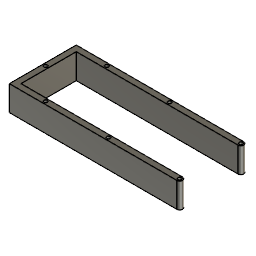
Belt Drive Arm (Autodesk Fusion 360 archive; units mm, degrees)
design "Wall"
Autodesk Fusion 360 part; units mm, degrees
sketch "Sketch1" plane through (0, 0, 0) normal (0, 0, 1) x (1, 0, 0)
  line L0 (0, 0) -> (160, 0)
  line L1 (0, 80) -> (160, 80)
  line L2 (0, 7) -> (160, 7)
  line L3 (160, 73) -> (0, 73)
  line L4 (0, 80) -> (-40, 80)
  line L5 (-40, 80) -> (-40, 0)
  line L6 (-40, 0) -> (0, 0)
  line L7 (0, 73) -> (-33, 73)
  line L8 (-33, 73) -> (-33, 7)
  line L9 (-33, 7) -> (0, 7)
  arc A0 (160, 73) -> (160, 80) centre (160, 76.5) ccw
  arc A1 (160, 0) -> (160, 7) centre (160, 3.5) ccw
  point P0 (0, 7)
  point P1 (0, 73)
  point P2 (160, 73)
  point P3 (160, 7)
  dimension "d1" = 160
  dimension "d2" = 80
  dimension "d3" = 7
  dimension "d4" = 7
  dimension "d5" = 7
  dimension "d6" = 7
  constraint coincident L0.start L6.end
  constraint horizontal L0
  constraint parallel L0 L1
  constraint coincident P0 L2.start
  constraint coincident P3 L2.end
  constraint parallel L0 L2
  constraint coincident P2 L3.start
  constraint coincident P1 L3.end
  constraint parallel L1 L4
  constraint perpendicular L1 L5
  constraint parallel L3 L7
  constraint perpendicular L2 L8
  constraint tangent L1 A0
  constraint tangent L0 A1
  measures "d1" distance of L0.start L0.end
  measures "d2" distance of L0 L1
  measures "d3" distance of L1.start P1
  measures "d4" distance of L0.start L2.start
  measures "d5" distance of L0.end P3
  measures "d6" distance of L1.end P2
extrude "Extrude1" add sketch "Sketch1" along normal blind 30
sketch "Sketch2" plane through (0, 0, 30) normal (0, 0, 1) x (-1, 0, 0)
  line L0 (40, 0) -> (-160, 0)
  line L1 (-160, -80) -> (40, -80)
  circle A0 centre (0, -3.5) radius 2.1
  circle A1 centre (0, -76.5) radius 2.1
  circle A2 centre (-160, -3.5) radius 2.1
  circle A3 centre (-160, -76.5) radius 2.1
  circle A4 centre (-75, -3.5) radius 2.1
  circle A5 centre (-75, -76.5) radius 2.1
  circle A6 centre (36.5, -40) radius 2.1
  line L2 (40, -80) -> (40, 0)
  line L3 (-160, -7) -> (33, -7)
  line L4 (33, -7) -> (33, -73)
  line L5 (33, -73) -> (-160, -73)
  arc A7 (-160, 0) -> (-160, -7) centre (-160, -3.5) ccw
  arc A8 (-160, -73) -> (-160, -80) centre (-160, -76.5) ccw
  point P0 (40, -40)
  point P1 (-75, -80)
  dimension "d9" = 4.2
  dimension "d10" = 4.2
  dimension "d11" = 4.2
  dimension "d12" = 4.2
  dimension "d13" = 4.2
  dimension "d14" = 4.2
  dimension "d15" = 4.2
  dimension "d21" = 3.5
  dimension "d22" = 3.5
  dimension "d23" = 3.5
  dimension "d24" = 3.5
  dimension "d28" = 85
  dimension "d29" = 85
  constraint coincident L1 P1
  measures "d9" diameter of A0
  measures "d10" diameter of A1
  measures "d11" diameter of A2
  measures "d12" diameter of A3
  measures "d13" diameter of A4
  measures "d14" diameter of A5
  measures "d15" diameter of A6
  measures "d21" distance of P0 A6.centre
  measures "d22" distance of L0 A0.centre
  measures "d23" distance of L0 A4.centre
  measures "d24" distance of L0 A2.centre
  measures "d28" horizontal distance of A3.centre P1
  measures "d29" horizontal distance of A2.centre P1
extrude "Extrude2" cut sketch "Sketch2" against normal blind 30 contours A0 | A1 | A2 | A3 | A4 | A5 | A6

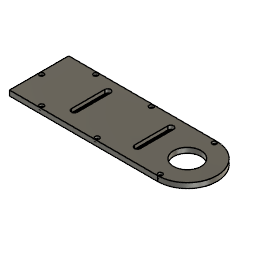
design "Top"
Autodesk Fusion 360 part; units mm, degrees
sketch "Sketch1" plane through (0, 0, 0) normal (0, 0, 1) x (1, 0, 0)
  line L0 (160, 80) -> (0, 80)
  line L1 (0, 0) -> (160, 0)
  arc A0 (160, 0) -> (160, 80) centre (160, 40) ccw
  line L2 (0, 80) -> (-40, 80)
  line L3 (-40, 80) -> (-40, 0)
  line L4 (-40, 0) -> (0, 0)
  dimension "d24" = 160
  dimension "d53" = 80
  constraint horizontal L0
  constraint coincident L1.start L4.end
  constraint tangent L1 A0
  constraint vertical L1.end L0.start
  constraint parallel L0 L2
  constraint perpendicular L2 L3
  measures "d24" distance of L1.start L1.end
  measures "d53" distance of L0 L1
extrude "Extrude1" add sketch "Sketch1" along normal blind 7
sketch "Sketch3" plane through (0, 0, 7) normal (0, 0, 1) x (-1, 0, 0)
  line L0 (40, 0) -> (-160, 0)
  line L1 (-160, -80) -> (40, -80)
  circle A0 centre (-75, -40) radius 3.05
  circle A1 centre (-75, -40) radius 5
  arc A2 (-160, 0) -> (-160, -80) centre (-160, -40) ccw
  line L2 (40, -80) -> (40, 0)
  point P0 (40, -40)
  dimension "d17" = 6.1
  dimension "d54" = 40
  dimension "d55" = 115
  constraint concentric A0 A1
  measures "d17" diameter of A0
  measures "d54" distance of L0 A0.centre
  measures "d55" distance of A0.centre P0
extrude "Extrude3" add sketch "Sketch3" against normal blind 8.7 contours A1
sketch "Sketch4" plane through (0, 0, 7) normal (0, 0, 1) x (-1, 0, 0)
  line L0 (40, 0) -> (-160, 0)
  line L1 (-160, -80) -> (40, -80)
  circle A0 centre (-160, -40) radius 18.5
  arc A1 (-160, 0) -> (-160, -80) centre (-160, -40) ccw
  line L2 (40, -80) -> (40, 0)
  point P0 (-200, -40)
  dimension "d25" = 37
  dimension "d56" = 40
  dimension "d57" = 40
  constraint midpoint A1 P0
  measures "d25" diameter of A0
  measures "d56" distance of L0 A0.centre
  measures "d57" distance of A0.centre P0
extrude "Extrude4" cut sketch "Sketch4" against normal blind 7 contours A0
sketch "Sketch7" plane through (0, 0, 7) normal (0, 0, 1) x (-1, 0, 0)
  circle A0 centre (-160, -40) radius 18.5
  arc A1 (-160, 0) -> (-160, -80) centre (-160, -40) ccw
  line L0 (-160, -80) -> (40, -80)
  line L1 (40, 0) -> (-160, 0)
  circle A2 centre (0, -76.5) radius 1.65
  circle A3 centre (0, -3.5) radius 1.65
  circle A4 centre (36.5, -40) radius 1.65
  circle A5 centre (-160, -76.5) radius 1.65
  circle A6 centre (-160, -3.5) radius 1.65
  circle A7 centre (-75, -3.5) radius 1.65
  circle A8 centre (-75, -76.5) radius 1.65
  line L2 (40, -80) -> (40, 0)
  point P0 (40, -40)
  point P1 (-75, -80)
  dimension "d58" = 3.3
  dimension "d59" = 3.3
  dimension "d60" = 3.3
  dimension "d62" = 3.3
  dimension "d63" = 3.3
  dimension "d64" = 3.3
  dimension "d65" = 3.3
  dimension "d66" = 3.5
  dimension "d68" = 3.5
  dimension "d69" = 3.5
  dimension "d70" = 3.5
  dimension "d73" = 3.5
  dimension "d86" = 3.5
  dimension "d87" = 85
  dimension "d88" = 85
  dimension "d106" = 40
  dimension "d107" = 3.5
  constraint coincident L0 P1
  measures "d58" diameter of A2
  measures "d59" diameter of A3
  measures "d60" diameter of A4
  measures "d62" diameter of A5
  measures "d63" diameter of A6
  measures "d64" diameter of A7
  measures "d65" diameter of A8
  measures "d66" distance of L0 A8.centre
  measures "d68" distance of L0 A5.centre
  measures "d69" distance of origin A3.centre
  measures "d70" distance of L1 A7.centre
  measures "d73" distance of P0 A4.centre
  measures "d86" distance of L1 A6.centre
  measures "d87" horizontal distance of A5.centre P1
  measures "d88" horizontal distance of A6.centre P1
  measures "d106" distance of A2.centre L2
  measures "d107" distance of L0 A2.centre
extrude "Extrude7" cut sketch "Sketch7" against normal blind 7 contours A2 | A3 | A4 | A5 | A6 | A7 | A8
sketch "Sketch8" plane through (0, 0, 7) normal (0, 0, 1) x (-1, 0, 0)
  circle A0 centre (-75, -76.5) radius 1.65
  circle A1 centre (-75, -3.5) radius 1.65
  circle A2 centre (36.5, -40) radius 1.65
  circle A3 centre (-160, -76.5) radius 1.65
  circle A4 centre (0, -3.5) radius 1.65
  circle A5 centre (-160, -40) radius 18.5
  arc A6 (-160, 0) -> (-160, -80) centre (-160, -40) ccw
  line L0 (-160, -80) -> (40, -80)
  line L1 (40, 0) -> (-160, 0)
  circle A7 centre (0, -76.5) radius 3
  circle A8 centre (36.5, -40) radius 3
  circle A9 centre (0, -3.5) radius 3
  circle A10 centre (-75, -76.5) radius 3
  circle A11 centre (-75, -3.5) radius 3
  circle A12 centre (-160, -76.5) radius 3
  circle A13 centre (-160, -3.5) radius 3
  circle A14 centre (-160, -3.5) radius 1.65
  line L2 (40, -80) -> (40, 0)
  circle A15 centre (0, -76.5) radius 1.65
  dimension "d76" = 6
  dimension "d77" = 6
  dimension "d78" = 6
  dimension "d79" = 6
  dimension "d80" = 6
  dimension "d81" = 6
  dimension "d82" = 6
  constraint concentric A7 A15
  constraint concentric A2 A8
  constraint concentric A4 A9
  constraint concentric A0 A10
  constraint concentric A1 A11
  constraint concentric A3 A12
  constraint concentric A13 A14
  measures "d76" diameter of A7
  measures "d77" diameter of A8
  measures "d78" diameter of A9
  measures "d79" diameter of A10
  measures "d80" diameter of A11
  measures "d81" diameter of A12
  measures "d82" diameter of A13
extrude "Extrude8" cut sketch "Sketch8" against normal blind 3 contours A7 | A8 | A9 | A10 | A11 | A12 | A13
sketch "Sketch9" plane through (0, 0, 7) normal (0, 0, 1) x (-1, 0, 0)
  circle A0 centre (-160, -76.5) radius 3
  circle A1 centre (36.5, -40) radius 3
  circle A2 centre (0, -3.5) radius 3
  circle A3 centre (-75, -76.5) radius 3
  circle A4 centre (-75, -3.5) radius 3
  circle A5 centre (-160, -3.5) radius 3
  circle A6 centre (-160, -40) radius 18.5
  arc A7 (-160, 0) -> (-160, -80) centre (-160, -40) ccw
  line L0 (-160, -80) -> (40, -80)
  line L1 (40, 0) -> (-160, 0)
  line L2 (-25, -20) -> (-25, -65)
  line L3 (-30.3, -20) -> (-30.3, -65)
  arc A8 (-30.3, -65) -> (-25, -65) centre (-27.65, -65) ccw
  arc A9 (-25, -20) -> (-30.3, -20) centre (-27.65, -20) ccw
  line L4 (-110, -20) -> (-110, -65)
  line L5 (-115.3, -20) -> (-115.3, -65)
  arc A10 (-110, -20) -> (-115.3, -20) centre (-112.65, -20) ccw
  arc A11 (-115.3, -65) -> (-110, -65) centre (-112.65, -65) ccw
  line L6 (40, -80) -> (40, 0)
  circle A12 centre (0, -76.5) radius 3
  point P0 (40, -40)
  point P1 (-160, -40)
  point P2 (-75, -40)
  dimension "d89" = 45
  dimension "d90" = 65
  dimension "d91" = 20
  dimension "d92" = 5.3
  dimension "d95" = 85
  dimension "d96" = 45
  dimension "d97" = 35
  dimension "d98" = 20
  dimension "d99" = 5.3
  constraint vertical L2
  constraint vertical L3
  constraint tangent L2 A8
  constraint tangent L3 A8
  constraint tangent L2 A9
  constraint coincident P1 A6.centre
  constraint vertical L4
  constraint vertical L5
  constraint tangent L4 A10
  constraint tangent L4 A11
  constraint tangent L5 A11
  measures "d89" distance of L2.start L2.end
  measures "d90" distance of P0 L2
  measures "d91" distance of L1 L2.start
  measures "d92" distance of L2 L3
  measures "d95" distance of P1 P2
  measures "d96" distance of L4.start L4.end
  measures "d97" distance of P2 L4
  measures "d98" distance of L1 L4.start
  measures "d99" distance of L4 L5
extrude "Extrude9" cut sketch "Sketch9" against normal blind 7 contours L2 L3 A8 A9 | L4 L5 A10 A11
sketch "Sketch10" plane through (0, 0, 7) normal (0, 0, 1) x (-1, 0, 0)
  line L0 (-30.3, -65) -> (-30.3, -20)
  arc A0 (-25, -20) -> (-30.3, -20) centre (-27.65, -20) ccw
  line L1 (-25, -20) -> (-25, -65)
  arc A1 (-30.3, -65) -> (-25, -65) centre (-27.65, -65) ccw
  line L2 (-115.3, -65) -> (-115.3, -20)
  arc A2 (-110, -20) -> (-115.3, -20) centre (-112.65, -20) ccw
  line L3 (-110, -20) -> (-110, -65)
  arc A3 (-115.3, -65) -> (-110, -65) centre (-112.65, -65) ccw
  circle A4 centre (-160, -76.5) radius 3
  circle A5 centre (36.5, -40) radius 3
  circle A6 centre (0, -3.5) radius 3
  circle A7 centre (-75, -76.5) radius 3
  circle A8 centre (-75, -3.5) radius 3
  circle A9 centre (-160, -3.5) radius 3
  circle A10 centre (-160, -40) radius 18.5
  arc A11 (-160, 0) -> (-160, -80) centre (-160, -40) ccw
  line L4 (-160, -80) -> (40, -80)
  line L5 (40, 0) -> (-160, 0)
  line L6 (-23.65, -20) -> (-23.65, -65)
  line L7 (-31.65, -20) -> (-31.65, -65)
  arc A12 (-31.65, -65) -> (-23.65, -65) centre (-27.65, -65) ccw
  arc A13 (-23.65, -20) -> (-31.65, -20) centre (-27.65, -20) ccw
  line L8 (-108.65, -20) -> (-108.65, -65)
  line L9 (-116.65, -20) -> (-116.65, -65)
  arc A14 (-116.65, -65) -> (-108.65, -65) centre (-112.65, -65) ccw
  arc A15 (-108.65, -20) -> (-116.65, -20) centre (-112.65, -20) ccw
  line L10 (40, -80) -> (40, 0)
  circle A16 centre (0, -76.5) radius 3
  dimension "d100" = 1.35
  dimension "d101" = 1.35
  dimension "d102" = 1.35
  dimension "d103" = 1.35
  constraint perpendicular L4 L6
  constraint parallel L0 L7
  constraint tangent L6 A12
  constraint tangent L7 A12
  constraint tangent L6 A13
  constraint tangent L7 A13
  constraint vertical L8
  constraint tangent L8 A14
  constraint tangent L9 A14
  constraint tangent L8 A15
  constraint tangent L9 A15
  measures "d100" distance of L1 L6
  measures "d101" distance of L0 L7
  measures "d102" distance of L3 L8
  measures "d103" distance of L2 L9
extrude "Extrude10" cut sketch "Sketch10" against normal blind 5 contours L6 L7 A12 A13 | L8 L9 A14 A15
sketch "Sketch11" plane through (-40, 0, 0) normal (-1, 0, 0) x (0, -1, 0)
  line L0 (-80, 0) -> (0, 0)
  line L1 (0, 0) -> (0, 7)
  line L2 (0, 7) -> (-80, 7)
  line L3 (-80, 7) -> (-80, 0)
  circle A0 centre (-76.5, 3.5) radius 2.1
  circle A1 centre (-3.5, 3.5) radius 2.1
  dimension "d108" = 4.2
  dimension "d109" = 3.5
  dimension "d110" = 4.2
  dimension "d111" = 3.5
  measures "d108" diameter of A0
  measures "d109" distance of L3 A0.centre
  measures "d110" diameter of A1
  measures "d111" distance of L1 A1.centre
extrude "Extrude11" cut sketch "Sketch11" against normal blind 10 contours A0 | A1

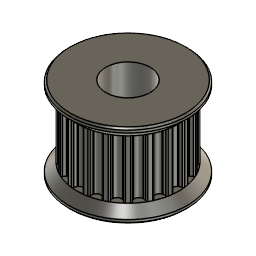
design "GT2-20"
Autodesk Fusion 360 part; units mm, degrees
sketch "Pulley Cylinder" plane through (0, 0, 0) normal (0, 0, 1) x (1, 0, 0) in component "Component"
  circle A0 centre (0, 0) radius 6.1122
extrude "Extrude1" add sketch "Pulley Cylinder" along normal blind 7 in component "Component"
ref_plane "WorkPlane1" through (0, 0, 7) normal (0, 0, 1) x (1, 0, 0) in component "Component"
sketch "Sketch2" plane through (0, 0, 7) normal (0, 0, 1) x (1, 0, 0) in component "Component"
  circle A0 centre (0, 0) radius 7.1122
ref_plane "WorkPlane2" through (0, 0, 0) normal (0, 0, 1) x (1, 0, 0) in component "Component"
sketch "Sketch3" plane through (0, 0, 0) normal (0, 0, 1) x (1, 0, 0) in component "Component"
  circle A0 centre (0, 0) radius 7.1122
extrude "Extrude2" add sketch "Sketch2" along normal blind 1.5 in component "Component"
extrude "Extrude3" add sketch "Sketch3" against normal blind 1.5 in component "Component"
chamfer "Chamfer1" distance 1 angle 45 1 edges at (-6.6309, -2.5719, 0) in component "Component"
chamfer "Chamfer2" distance 1 angle 45 1 edges at (-6.6309, -2.5719, 7) in component "Component"
chamfer "Chamfer3" distance 0.2 angle 45 1 edges at (-6.6309, 2.5719, -1.5) in component "Component"
chamfer "Chamfer4" distance 0.2 angle 45 1 edges at (-6.6309, -2.5719, 8.5) in component "Component"
sketch "Bore" plane through (0, 0, 0) normal (0, 0, 1) x (1, 0, 0) in component "Component"
  circle A0 centre (0, 0) radius 2.65
  constraint coincident A0.centre origin
extrude "Extrude4" cut sketch "Bore" along normal blind 8.5 and the other way blind 1.5 in component "Component"
sketch "Tooth Profile" plane through (0, 0, 0) normal (0, 0, 1) x (1, 0, 0) in component "Component"
  circle A0 centre (0, 0) radius 6.1122 construction
  line L0 (-9.1683, 0) -> (9.1683, 0) construction
  line L1 (6.1122, -6.1122) -> (6.1122, 6.1122) construction
  line L2 (5.1981, 0.4143) -> (6.0981, 0.4143) construction
  line L3 (5.1981, -0.4143) -> (6.0981, -0.4143) construction
  arc A1 (5.5489, 0.4143) -> (5.5489, -0.4143) centre (5.9153, 0) ccw
  line L4 (5.3622, 0.4) -> (5.3622, -0.4) construction
  line L5 (5.5489, 0.4143) -> (5.5489, -0.4143) construction
  arc A2 (5.6176, -0.4626) -> (5.9418, -0.5734) centre (6.0981, 0.4143) ccw
  arc A3 (5.9418, 0.5734) -> (5.6176, 0.4626) centre (6.0981, -0.4143) ccw
  arc A4 (5.9418, 0.5734) -> (6.0673, 0.7397) centre (5.9184, 0.7215) ccw
  arc A5 (5.6176, 0.4626) -> (5.5489, 0.4143) centre (5.799, 0.1316) ccw
  arc A6 (6.0673, -0.7397) -> (5.9418, -0.5734) centre (5.9184, -0.7215) ccw
  arc A7 (5.5489, -0.4143) -> (5.6176, -0.4626) centre (5.799, -0.1316) ccw
  arc A8 (6.0673, -0.7397) -> (6.0673, 0.7397) centre (0, 0) ccw
  point P0 (5.9153, 0)
  point P1 (5.9172, 0)
  point P2 (5.9172, 0)
  dimension "d17" = 12.2244
  dimension "d18" = 0.8287
  dimension "d19" = 0.75
  dimension "d20" = 0.5633
  dimension "d21" = 1
  dimension "d22" = 1
  dimension "d23" = 0.15
  dimension "d24" = 0.15
  constraint coincident A0 L2.end
  constraint coincident A0 L3.end
  constraint coincident A0.centre A8.centre
  constraint midpoint A0.centre L0
  constraint horizontal L0
  constraint vertical L1
  constraint tangent A0 L1
  constraint symmetric L0 L2.start L3.start
  constraint symmetric L0 L2.end L3.end
  constraint horizontal L2
  constraint coincident L2 A1.start
  constraint coincident L3 A1.end
  constraint coincident P0 A1.centre
  constraint symmetric L0 A1.start A1.end
  constraint vertical L4
  constraint tangent A1 L4
  constraint coincident L2.end A2.centre
  constraint coincident L3.end A3.centre
  constraint coincident A0 A4.end
  constraint coincident A3.start A4.start
  constraint tangent A3 A4
  constraint tangent A0 A4
  constraint tangent A1 A5
  constraint coincident A3.end A5.start
  constraint tangent A3 A5
  constraint coincident A0 A6.start
  constraint coincident A2.end A6.end
  constraint tangent A2 A6
  constraint tangent A0 A6
  constraint tangent A1 A7
  constraint coincident A2.start A7.end
  constraint tangent A2 A7
  constraint coincident A4.end A8.end
  measures "d17" diameter of A0
  measures "d18" vertical distance of L2.start L3.start
  measures "d19" horizontal distance of L1.start L4.start
  measures "d20" horizontal distance of L1.start A1.start
  measures "d21" radius of A2
  measures "d22" radius of A3
  measures "d23" radius of A4
  measures "d24" radius of A6
extrude "Extrude5" cut sketch "Tooth Profile" along normal blind 7 in component "Component"
pattern_circular "C-Pattern1" count 20 over 360 about axis through (0, 0, 1.75) along (0, 0, 1) of "Extrude5" in component "Component"
component "Component" placed x (1, 0, 0) y (0, 1, 0) z (0, 0, 1) at (0, 0, 0)
named bodies: "GT2 Pulley"

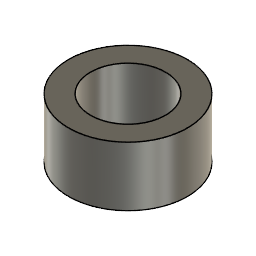
design "Spacer 5mm"
Autodesk Fusion 360 part; units mm, degrees
sketch "Sketch1" plane through (0, 0, 0) normal (0, 0, 1) x (1, 0, 0)
  circle A0 centre (0, 0) radius 3.15
  circle A1 centre (0, 0) radius 5
  dimension "d1" = 6.3
  dimension "d2" = 10
  constraint coincident A0.centre A1.centre
  constraint concentric A0 A1
  measures "d1" diameter of A0
  measures "d2" diameter of A1
extrude "Extrude1" add sketch "Sketch1" along normal blind 5

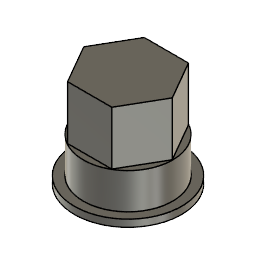
design "Pin"
Autodesk Fusion 360 part; units mm, degrees
sketch "Sketch1" plane through (0, 0, 0) normal (0, 0, 1) x (1, 0, 0)
  circle A0 centre (0, 0) radius 12.5
  dimension "d1" = 25
  constraint coincident A0.centre origin
  measures "d1" diameter of A0
extrude "Extrude1" add sketch "Sketch1" along normal blind 10
sketch "Sketch2" plane through (0, 0, 10) normal (0, 0, 1) x (-1, 0, 0)
  circle A0 centre (0, 0) radius 12.5
  line L0 (-12.4, 0) -> (-6.2, -10.7387)
  line L1 (-6.2, -10.7387) -> (6.2, -10.7387)
  line L2 (6.2, -10.7387) -> (12.4, 0)
  line L3 (12.4, 0) -> (6.2, 10.7387)
  line L4 (6.2, 10.7387) -> (-6.2, 10.7387)
  line L5 (-6.2, 10.7387) -> (-12.4, 0)
  dimension "d9" = 12.4
  constraint coincident A0.centre origin
  measures "d9" distance of L0.start A0.centre
extrude "Extrude2" add sketch "Sketch2" along normal blind 15 contours L0 L1 L2 L3 L4 L5
sketch "Sketch3" plane through (0, 0, 0) normal (0, 0, -1) x (1, 0, 0)
  circle A0 centre (0, 0) radius 12.5
  circle A1 centre (0, 0) radius 15
  dimension "d6" = 30
  constraint coincident A0.centre A1.centre
  measures "d6" diameter of A1
extrude "Extrude3" add sketch "Sketch3" along normal blind 2 contours A0 | A1

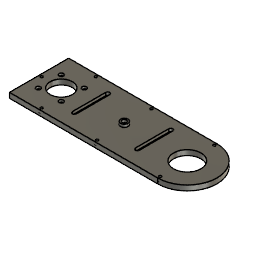
design "Base"
Autodesk Fusion 360 part; units mm, degrees
sketch "Sketch1" plane through (0, 0, 0) normal (0, 0, 1) x (1, 0, 0)
  line L0 (160, 80) -> (0, 80)
  line L1 (0, 0) -> (160, 0)
  arc A0 (160, 0) -> (160, 80) centre (160, 40) ccw
  line L2 (0, 80) -> (-40, 80)
  line L3 (-40, 80) -> (-40, 0)
  line L4 (-40, 0) -> (0, 0)
  dimension "d24" = 160
  dimension "d53" = 80
  constraint horizontal L0
  constraint coincident L1.start L4.end
  constraint tangent L1 A0
  constraint tangent L0 A0
  constraint parallel L0 L2
  constraint perpendicular L0 L3
  measures "d24" distance of L1.start L1.end
  measures "d53" distance of L0 L1
extrude "Extrude1" add sketch "Sketch1" along normal blind 7
sketch "Sketch2" plane through (0, 0, 7) normal (0, 0, 1) x (-1, 0, 0)
  line L0 (40, 0) -> (-160, 0)
  line L1 (-160, -80) -> (40, -80)
  circle A0 centre (10, -40) radius 15
  circle A1 centre (25.5, -55.5) radius 1.65
  circle A2 centre (25.5, -24.5) radius 1.65
  circle A3 centre (-5.5, -55.5) radius 1.65
  circle A4 centre (-5.5, -24.5) radius 1.65
  arc A5 (-160, 0) -> (-160, -80) centre (-160, -40) ccw
  line L2 (40, -80) -> (40, 0)
  point P0 (40, -40)
  dimension "d4" = 30
  dimension "d5" = 3.3
  dimension "d6" = 15.5
  dimension "d7" = 15.5
  dimension "d8" = 3.3
  dimension "d9" = 15.5
  dimension "d10" = 3.3
  dimension "d11" = 15.5
  dimension "d12" = 3.3
  dimension "d55" = 15.5
  dimension "d58" = 30
  dimension "d59" = 40
  dimension "d60" = 15.5
  dimension "d61" = 15.5
  dimension "d128" = 15.5
  measures "d4" diameter of A0
  measures "d5" diameter of A1
  measures "d6" vertical distance of A0.centre A1.centre
  measures "d7" horizontal distance of A0.centre A1.centre
  measures "d8" diameter of A2
  measures "d9" vertical distance of A0.centre A2.centre
  measures "d10" diameter of A3
  measures "d11" horizontal distance of A0.centre A3.centre
  measures "d12" diameter of A4
  measures "d55" vertical distance of A0.centre A4.centre
  measures "d58" distance of A0.centre P0
  measures "d59" distance of L0 A0.centre
  measures "d60" horizontal distance of A0.centre A2.centre
  measures "d61" horizontal distance of A0.centre A4.centre
  measures "d128" vertical distance of A0.centre A3.centre
extrude "Extrude2" cut sketch "Sketch2" against normal blind 10 contours A0 | A1 | A2 | A3 | A4
sketch "Sketch3" plane through (0, 0, 7) normal (0, 0, 1) x (-1, 0, 0)
  circle A0 centre (25.5, -24.5) radius 1.65
  circle A1 centre (-5.5, -24.5) radius 1.65
  circle A2 centre (-5.5, -55.5) radius 1.65
  circle A3 centre (10, -40) radius 15
  circle A4 centre (25.5, -55.5) radius 1.65
  line L0 (40, 0) -> (-160, 0)
  line L1 (-160, -80) -> (40, -80)
  circle A5 centre (-75, -40) radius 3.05
  circle A6 centre (-75, -40) radius 5
  arc A7 (-160, 0) -> (-160, -80) centre (-160, -40) ccw
  line L2 (40, -80) -> (40, 0)
  point P0 (-200, -40)
  dimension "d17" = 6.1
  dimension "d18" = 85
  dimension "d56" = 40
  constraint concentric A5 A6
  constraint midpoint A7 P0
  measures "d17" diameter of A5
  measures "d18" distance of A3.centre A5.centre
  measures "d56" distance of L0 A5.centre
extrude "Extrude3" add sketch "Sketch3" along normal blind 3.7 contours A6
sketch "Sketch7" plane through (0, 0, 0) normal (0, 0, -1) x (1, 0, 0)
  circle A0 centre (-25.5, -24.5) radius 1.65
  circle A1 centre (5.5, -24.5) radius 1.65
  circle A2 centre (5.5, -55.5) radius 1.65
  circle A3 centre (-10, -40) radius 15
  circle A4 centre (-25.5, -55.5) radius 1.65
  arc A5 (160, -80) -> (160, 0) centre (160, -40) ccw
  line L0 (160, 0) -> (-40, 0)
  line L1 (-40, -80) -> (160, -80)
  circle A6 centre (0, -76.5) radius 1.65
  circle A7 centre (0, -3.5) radius 1.65
  circle A8 centre (160, -3.5) radius 1.65
  circle A9 centre (160, -76.5) radius 1.65
  circle A10 centre (75, -3.5) radius 1.65
  circle A11 centre (75, -76.5) radius 1.65
  circle A12 centre (-36.5, -40) radius 1.65
  line L2 (-40, 0) -> (-40, -80)
  point P0 (-40, -40)
  point P1 (75, -80)
  dimension "d62" = 3.3
  dimension "d63" = 3.5
  dimension "d64" = 3.3
  dimension "d66" = 3.3
  dimension "d68" = 3.3
  dimension "d70" = 3.3
  dimension "d71" = 3.3
  dimension "d72" = 3.5
  dimension "d73" = 3.5
  dimension "d76" = 3.3
  dimension "d77" = 3.5
  dimension "d90" = 3.5
  dimension "d91" = 3.5
  dimension "d92" = 85
  dimension "d93" = 85
  dimension "d116" = 40
  dimension "d117" = 3.5
  constraint coincident L1 P1
  measures "d62" diameter of A6
  measures "d63" distance of L1 A6.centre
  measures "d64" diameter of A7
  measures "d66" diameter of A8
  measures "d68" diameter of A9
  measures "d70" diameter of A10
  measures "d71" diameter of A11
  measures "d72" distance of L0 A10.centre
  measures "d73" distance of L1 A11.centre
  measures "d76" diameter of A12
  measures "d77" distance of P0 A12.centre
  measures "d90" distance of L0 A8.centre
  measures "d91" distance of L1 A9.centre
  measures "d92" horizontal distance of A9.centre P1
  measures "d93" horizontal distance of A8.centre P1
  measures "d116" distance of A7.centre L2
  measures "d117" distance of L0 A7.centre
extrude "Extrude7" cut sketch "Sketch7" against normal blind 7 contours A6 | A7 | A8 | A9 | A10 | A11 | A12
sketch "Sketch8" plane through (0, 0, 0) normal (0, 0, -1) x (1, 0, 0)
  circle A0 centre (75, -76.5) radius 1.65
  circle A1 centre (75, -3.5) radius 1.65
  circle A2 centre (160, -3.5) radius 1.65
  circle A3 centre (0, -76.5) radius 1.65
  circle A4 centre (160, -76.5) radius 1.65
  circle A5 centre (-36.5, -40) radius 1.65
  circle A6 centre (-25.5, -24.5) radius 1.65
  circle A7 centre (5.5, -24.5) radius 1.65
  circle A8 centre (5.5, -55.5) radius 1.65
  circle A9 centre (-10, -40) radius 15
  circle A10 centre (-25.5, -55.5) radius 1.65
  arc A11 (160, -80) -> (160, 0) centre (160, -40) ccw
  line L0 (160, 0) -> (-40, 0)
  line L1 (-40, -80) -> (160, -80)
  circle A12 centre (0, -3.5) radius 3
  circle A13 centre (-36.5, -40) radius 3
  circle A14 centre (0, -76.5) radius 3
  circle A15 centre (75, -3.5) radius 3
  circle A16 centre (75, -76.5) radius 3
  circle A17 centre (160, -3.5) radius 3
  circle A18 centre (160, -76.5) radius 3
  line L2 (-40, 0) -> (-40, -80)
  circle A19 centre (0, -3.5) radius 1.65
  dimension "d80" = 6
  dimension "d81" = 6
  dimension "d82" = 6
  dimension "d83" = 6
  dimension "d84" = 6
  dimension "d85" = 6
  dimension "d86" = 6
  constraint concentric A12 A19
  constraint concentric A5 A13
  constraint concentric A3 A14
  constraint concentric A1 A15
  constraint concentric A0 A16
  constraint concentric A2 A17
  constraint concentric A4 A18
  measures "d80" diameter of A12
  measures "d81" diameter of A13
  measures "d82" diameter of A14
  measures "d83" diameter of A15
  measures "d84" diameter of A16
  measures "d85" diameter of A17
  measures "d86" diameter of A18
extrude "Extrude8" cut sketch "Sketch8" against normal blind 3 contours A12 | A13 | A14 | A15 | A16 | A17 | A18
sketch "Sketch9" plane through (0, 0, 7) normal (0, 0, 1) x (-1, 0, 0)
  circle A0 centre (-75, -40) radius 5
  circle A1 centre (25.5, -24.5) radius 1.65
  circle A2 centre (-5.5, -24.5) radius 1.65
  circle A3 centre (-5.5, -55.5) radius 1.65
  circle A4 centre (10, -40) radius 15
  circle A5 centre (25.5, -55.5) radius 1.65
  arc A6 (-160, 0) -> (-160, -80) centre (-160, -40) ccw
  line L0 (-160, -80) -> (40, -80)
  line L1 (40, 0) -> (-160, 0)
  line L2 (-25, -20) -> (-25, -65)
  line L3 (-30.3, -20) -> (-30.3, -65)
  arc A7 (-30.3, -65) -> (-25, -65) centre (-27.65, -65) ccw
  arc A8 (-25, -20) -> (-30.3, -20) centre (-27.65, -20) ccw
  line L4 (-110, -20) -> (-110, -65)
  line L5 (-115.3, -20) -> (-115.3, -65)
  arc A9 (-110, -20) -> (-115.3, -20) centre (-112.65, -20) ccw
  arc A10 (-115.3, -65) -> (-110, -65) centre (-112.65, -65) ccw
  line L6 (40, -80) -> (40, 0)
  circle A11 centre (-75, -76.5) radius 1.65
  circle A12 centre (-75, -3.5) radius 1.65
  circle A13 centre (-160, -3.5) radius 1.65
  circle A14 centre (0, -76.5) radius 1.65
  circle A15 centre (-160, -76.5) radius 1.65
  circle A16 centre (0, -3.5) radius 1.65
  circle A17 centre (36.5, -40) radius 1.65
  dimension "d94" = 45
  dimension "d95" = 35
  dimension "d96" = 20
  dimension "d97" = 5.3
  dimension "d100" = 35
  dimension "d101" = 20
  dimension "d102" = 5.3
  constraint perpendicular L1 L2
  constraint vertical L3
  constraint tangent L2 A7
  constraint tangent L2 A8
  constraint tangent L3 A8
  constraint vertical L4
  constraint vertical L5
  constraint tangent L4 A9
  constraint tangent L4 A10
  constraint tangent L5 A10
  measures "d94" distance of L2.start L2.end
  measures "d95" distance of A4.centre L2
  measures "d96" distance of L1 L2.start
  measures "d97" distance of L2 L3
  measures "d100" distance of A0.centre L4
  measures "d101" distance of L1 L4.start
  measures "d102" distance of L4 L5
extrude "Extrude9" cut sketch "Sketch9" against normal blind 5 contours L2 L3 A7 A8 | L4 L5 A9 A10
sketch "Sketch10" plane through (0, 0, 0) normal (0, 0, -1) x (1, 0, 0)
  circle A0 centre (160, -76.5) radius 3
  circle A1 centre (-36.5, -40) radius 3
  circle A2 centre (0, -76.5) radius 3
  circle A3 centre (160, -3.5) radius 3
  circle A4 centre (75, -76.5) radius 3
  circle A5 centre (75, -3.5) radius 3
  circle A6 centre (-25.5, -24.5) radius 1.65
  circle A7 centre (5.5, -24.5) radius 1.65
  circle A8 centre (5.5, -55.5) radius 1.65
  circle A9 centre (-10, -40) radius 15
  circle A10 centre (-25.5, -55.5) radius 1.65
  arc A11 (160, -80) -> (160, 0) centre (160, -40) ccw
  line L0 (160, 0) -> (-40, 0)
  line L1 (-40, -80) -> (160, -80)
  line L2 (22.65, -65) -> (22.65, -20)
  line L3 (32.65, -65) -> (32.65, -20)
  arc A12 (32.65, -20) -> (22.65, -20) centre (27.65, -20) ccw
  arc A13 (22.65, -65) -> (32.65, -65) centre (27.65, -65) ccw
  line L4 (107.65, -65) -> (107.65, -20)
  line L5 (117.65, -65) -> (117.65, -20)
  arc A14 (117.65, -20) -> (107.65, -20) centre (112.65, -20) ccw
  arc A15 (107.65, -65) -> (117.65, -65) centre (112.65, -65) ccw
  line L6 (-40, 0) -> (-40, -80)
  circle A16 centre (0, -3.5) radius 3
  dimension "d103" = 45
  constraint perpendicular L1 L2
  constraint tangent L2 A12
  constraint tangent L2 A13
  constraint tangent L3 A13
  constraint tangent L4 A14
  constraint tangent L5 A14
  constraint tangent L4 A15
  constraint tangent L5 A15
  measures "d103" distance of L2.start L2.end
extrude "Extrude10" cut sketch "Sketch10" against normal blind 3 contours L2 L3 A12 A13 | L4 L5 A14 A15
sketch "Sketch11" plane through (0, 0, 7) normal (0, 0, 1) x (-1, 0, 0)
  line L0 (-30.3, -65) -> (-30.3, -20)
  arc A0 (-25, -20) -> (-30.3, -20) centre (-27.65, -20) ccw
  line L1 (-25, -20) -> (-25, -65)
  arc A1 (-30.3, -65) -> (-25, -65) centre (-27.65, -65) ccw
  line L2 (-115.3, -65) -> (-115.3, -20)
  arc A2 (-110, -20) -> (-115.3, -20) centre (-112.65, -20) ccw
  line L3 (-110, -20) -> (-110, -65)
  arc A3 (-115.3, -65) -> (-110, -65) centre (-112.65, -65) ccw
  circle A4 centre (-75, -40) radius 5
  circle A5 centre (25.5, -24.5) radius 1.65
  circle A6 centre (-5.5, -24.5) radius 1.65
  circle A7 centre (-5.5, -55.5) radius 1.65
  circle A8 centre (10, -40) radius 15
  circle A9 centre (25.5, -55.5) radius 1.65
  arc A10 (-160, 0) -> (-160, -80) centre (-160, -40) ccw
  line L4 (-160, -80) -> (40, -80)
  line L5 (40, 0) -> (-160, 0)
  circle A11 centre (-5.5, -55.5) radius 3
  circle A12 centre (25.5, -55.5) radius 3
  circle A13 centre (25.5, -24.5) radius 3
  circle A14 centre (-5.5, -24.5) radius 3
  line L6 (40, -80) -> (40, 0)
  circle A15 centre (-75, -76.5) radius 1.65
  circle A16 centre (-75, -3.5) radius 1.65
  circle A17 centre (-160, -3.5) radius 1.65
  circle A18 centre (0, -76.5) radius 1.65
  circle A19 centre (-160, -76.5) radius 1.65
  circle A20 centre (0, -3.5) radius 1.65
  circle A21 centre (36.5, -40) radius 1.65
  dimension "d110" = 6
  dimension "d111" = 6
  dimension "d112" = 6
  dimension "d113" = 6
  constraint concentric A7 A11
  constraint concentric A9 A12
  constraint concentric A5 A13
  constraint concentric A6 A14
  measures "d110" diameter of A11
  measures "d111" diameter of A12
  measures "d112" diameter of A13
  measures "d113" diameter of A14
extrude "Extrude11" cut sketch "Sketch11" against normal blind 3 contours A11 | A12 | A13 | A14
sketch "Sketch12" plane through (-40, 0, 0) normal (-1, 0, 0) x (0, -1, 0)
  line L0 (-80, 0) -> (0, 0)
  line L1 (0, 0) -> (0, 7)
  line L2 (0, 7) -> (-80, 7)
  line L3 (-80, 7) -> (-80, 0)
  circle A0 centre (-76.5, 3.5) radius 2.1
  circle A1 centre (-3.5, 3.5) radius 2.1
  dimension "d118" = 4.2
  dimension "d119" = 3.5
  dimension "d120" = 3.5
  dimension "d121" = 4.2
  dimension "d122" = 3.5
  measures "d118" diameter of A0
  measures "d119" distance of L2 A0.centre
  measures "d120" distance of L3 A0.centre
  measures "d121" diameter of A1
  measures "d122" distance of L1 A1.centre
extrude "Extrude12" cut sketch "Sketch12" against normal blind 10 contours A0 | A1
sketch "Sketch13" plane through (0, 0, 7) normal (0, 0, 1) x (-1, 0, 0)
  circle A0 centre (-5.5, -55.5) radius 3
  circle A1 centre (-5.5, -24.5) radius 3
  circle A2 centre (25.5, -55.5) radius 3
  circle A3 centre (25.5, -24.5) radius 3
  line L0 (-30.3, -65) -> (-30.3, -20)
  arc A4 (-25, -20) -> (-30.3, -20) centre (-27.65, -20) ccw
  line L1 (-25, -20) -> (-25, -65)
  arc A5 (-30.3, -65) -> (-25, -65) centre (-27.65, -65) ccw
  line L2 (-115.3, -65) -> (-115.3, -20)
  arc A6 (-110, -20) -> (-115.3, -20) centre (-112.65, -20) ccw
  line L3 (-110, -20) -> (-110, -65)
  arc A7 (-115.3, -65) -> (-110, -65) centre (-112.65, -65) ccw
  circle A8 centre (-75, -76.5) radius 1.65
  circle A9 centre (-75, -3.5) radius 1.65
  circle A10 centre (-160, -3.5) radius 1.65
  circle A11 centre (0, -76.5) radius 1.65
  circle A12 centre (-160, -76.5) radius 1.65
  circle A13 centre (0, -3.5) radius 1.65
  circle A14 centre (36.5, -40) radius 1.65
  line L4 (40, 0) -> (-160, 0)
  arc A15 (-160, 0) -> (-160, -80) centre (-160, -40) ccw
  line L5 (-160, -80) -> (40, -80)
  line L6 (40, -80) -> (40, 0)
  circle A16 centre (10, -40) radius 15
  circle A17 centre (-75, -40) radius 5
  circle A18 centre (-160, -40) radius 18.5
  dimension "d125" = 37
  constraint concentric A15 A18
  measures "d125" diameter of A18
extrude "Extrude13" cut sketch "Sketch13" against normal blind 7 contours A18

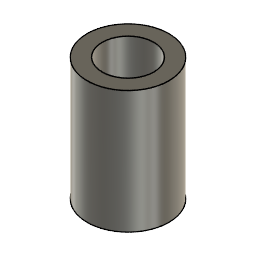
design "Spacer 15mm"
Autodesk Fusion 360 part; units mm, degrees
sketch "Sketch1" plane through (0, 0, 0) normal (0, 0, 1) x (1, 0, 0)
  circle A0 centre (0, 0) radius 3.15
  circle A1 centre (0, 0) radius 5
  dimension "d1" = 6.3
  dimension "d2" = 10
  constraint coincident A0.centre A1.centre
  constraint concentric A0 A1
  measures "d1" diameter of A0
  measures "d2" diameter of A1
extrude "Extrude1" add sketch "Sketch1" along normal blind 15

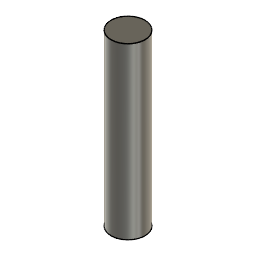
design "dowel pin 6x30mm"
Autodesk Fusion 360 part; units mm, degrees
sketch "Sketch1" plane through (0, 0, 0) normal (0, 0, 1) x (1, 0, 0)
  circle A0 centre (0, 0) radius 3
  dimension "d1" = 6
  constraint coincident A0.centre origin
  measures "d1" diameter of A0
extrude "Extrude1" add sketch "Sketch1" along normal blind 30

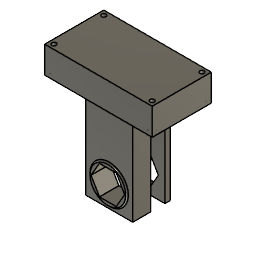
design "Output block"
Autodesk Fusion 360 part; units mm, degrees
sketch "Sketch1" plane through (0, 0, 0) normal (0, 1, 0) x (1, 0, 0)
  line L0 (0, 0) -> (35, 0)
  line L1 (35, 0) -> (35, -70)
  line L2 (35, -70) -> (0, -70)
  line L3 (0, -70) -> (0, 0)
  line L4 (30, -15.8253) -> (23.75, -5)
  line L5 (23.75, -5) -> (11.25, -5)
  line L6 (11.25, -5) -> (5, -15.8253)
  line L7 (5, -15.8253) -> (11.25, -26.6506)
  line L8 (11.25, -26.6506) -> (23.75, -26.6506)
  line L9 (23.75, -26.6506) -> (30, -15.8253)
  point P0 (17.5, -15.8253)
  dimension "d1" = 35
  dimension "d2" = 70
  dimension "d3" = 12.5
  dimension "d4" = 17.5
  dimension "d6" = 5
  constraint horizontal L0
  constraint vertical L1
  constraint horizontal L2
  constraint vertical L3
  constraint coincident L0.start L3.end
  constraint parallel L0 L5
  measures "d1" distance of L0.start L0.end
  measures "d2" distance of L0.start L2.end
  measures "d3" distance of L4.start P0
  measures "d4" distance of L3 P0
  measures "d6" distance of L0 L5
extrude "Extrude1" add sketch "Sketch1" along normal blind 28
sketch "Sketch2" plane through (35, 0, 0) normal (1, 0, 0) x (0, 1, 0)
  line L0 (0, 70) -> (0, 0)
  line L1 (0, 0) -> (28, 0)
  line L2 (28, 0) -> (28, 70)
  line L3 (28, 70) -> (0, 70)
  line L4 (13.5, 0) -> (24, 0)
  line L5 (24, 0) -> (24, 55)
  line L6 (24, 55) -> (13.5, 55)
  line L7 (13.5, 55) -> (13.5, 0)
  dimension "d9" = 10.5
  dimension "d10" = 55
  dimension "d14" = 4
  constraint horizontal L4
  constraint vertical L5
  constraint horizontal L6
  constraint vertical L7
  constraint coincident L1 L4.start
  measures "d9" distance of L4.start L4.end
  measures "d10" distance of L4.start L6.end
  measures "d14" distance of L2 L5
extrude "Extrude2" cut sketch "Sketch2" against normal blind 35 contours L1 L4 L5 L6 L7
sketch "Sketch3" plane through (0, 0, 70) normal (0, 0, 1) x (-1, 0, 0)
  line L0 (0, 0) -> (-35, 0)
  line L1 (-35, 0) -> (-35, -28)
  line L2 (-35, -28) -> (0, -28)
  line L3 (0, -28) -> (0, 0)
  line L4 (-57.5, -36) -> (22.5, -36)
  line L5 (22.5, -36) -> (22.5, 8)
  line L6 (22.5, 8) -> (-57.5, 8)
  line L7 (-57.5, 8) -> (-57.5, -36)
  dimension "d15" = 80
  dimension "d16" = 44
  dimension "d17" = 22.5
  dimension "d18" = 8
  constraint horizontal L4
  constraint vertical L5
  constraint horizontal L6
  constraint vertical L7
  measures "d15" distance of L4.start L4.end
  measures "d16" distance of L4.start L6.end
  measures "d17" distance of L3 L5
  measures "d18" distance of L0 L6
extrude "Extrude3" add sketch "Sketch3" along normal blind 20 contours L0 L1 L2 L3 | L4 L5 L6 L7
fillet "Fillet1" radius 5 4 edges at (17.5, 28, 70) (35, 14, 70) (17.5, 0, 70) (0, 14, 70)
sketch "Sketch4" plane through (0, 0, 70) normal (0, 0, -1) x (1, 0, 0)
  line L0 (57.5, -36) -> (57.5, 8)
  line L1 (57.5, 8) -> (-22.5, 8)
  line L2 (-22.5, 8) -> (-22.5, -36)
  line L3 (-22.5, -36) -> (57.5, -36)
  line L4 (-5, 5) -> (40, 5)
  line L5 (40, 5) -> (40, -33)
  line L6 (40, -33) -> (-5, -33)
  line L7 (-5, -33) -> (-5, 5)
  circle A0 centre (54, -32.5) radius 1.65
  circle A1 centre (54, 4.5) radius 1.65
  circle A2 centre (-19, -32.5) radius 1.65
  circle A3 centre (-19, 4.5) radius 1.65
  dimension "d23" = 3.3
  dimension "d24" = 3.5
  dimension "d25" = 3.5
  dimension "d26" = 3.3
  dimension "d27" = 3.5
  dimension "d28" = 3.3
  dimension "d29" = 3.5
  dimension "d30" = 3.3
  dimension "d31" = 3.5
  dimension "d32" = 3.5
  dimension "d33" = 3.5
  measures "d23" diameter of A0
  measures "d24" distance of L3 A0.centre
  measures "d25" distance of L0 A0.centre
  measures "d26" diameter of A1
  measures "d27" distance of L1 A1.centre
  measures "d28" diameter of A2
  measures "d29" distance of L2 A2.centre
  measures "d30" diameter of A3
  measures "d31" distance of L1 A3.centre
  measures "d32" distance of L3 A2.centre
  measures "d33" distance of L2 A3.centre
extrude "Extrude4" cut sketch "Sketch4" against normal blind 20 contours A0 | A1 | A2 | A3
sketch "Sketch5" plane through (0, 0, 70) normal (0, 0, -1) x (1, 0, 0)
  circle A0 centre (54, -32.5) radius 1.65
  circle A1 centre (54, 4.5) radius 1.65
  circle A2 centre (-19, -32.5) radius 1.65
  circle A3 centre (-19, 4.5) radius 1.65
  line L0 (57.5, -36) -> (57.5, 8)
  line L1 (57.5, 8) -> (-22.5, 8)
  line L2 (-22.5, 8) -> (-22.5, -36)
  line L3 (-22.5, -36) -> (57.5, -36)
  line L4 (-5, 5) -> (40, 5)
  line L5 (40, 5) -> (40, -33)
  line L6 (40, -33) -> (-5, -33)
  line L7 (-5, -33) -> (-5, 5)
  circle A4 centre (-19, -32.5) radius 3
  circle A5 centre (-19, 4.5) radius 3
  circle A6 centre (54, 4.5) radius 3
  circle A7 centre (54, -32.5) radius 3
  dimension "d36" = 6
  dimension "d37" = 6
  dimension "d38" = 6
  dimension "d39" = 6
  constraint concentric A2 A4
  constraint concentric A3 A5
  constraint concentric A1 A6
  constraint concentric A0 A7
  measures "d36" diameter of A4
  measures "d37" diameter of A5
  measures "d38" diameter of A6
  measures "d39" diameter of A7
extrude "Extrude5" cut sketch "Sketch5" against normal blind 3 contours A4 | A5 | A6 | A7
sketch "Sketch6" plane through (0, 0, 0) normal (0, -1, 0) x (1, 0, 0)
  line L0 (35, 65) -> (0, 65)
  line L1 (0, 65) -> (0, 0)
  line L2 (0, 0) -> (35, 0)
  line L3 (35, 0) -> (35, 65)
  line L4 (23.75, 26.6506) -> (30, 15.8253)
  line L5 (30, 15.8253) -> (23.75, 5)
  line L6 (23.75, 5) -> (11.25, 5)
  line L7 (11.25, 5) -> (5, 15.8253)
  line L8 (5, 15.8253) -> (11.25, 26.6506)
  line L9 (11.25, 26.6506) -> (23.75, 26.6506)
  circle A0 centre (17.5, 15.825) radius 13.25
  dimension "d42" = 26.5
  dimension "d43" = 15.825
  measures "d42" diameter of A0
  measures "d43" distance of L2 A0.centre
extrude "Extrude6" add sketch "Sketch6" along normal blind 1 contours A0
fillet "Fillet2" radius 1 1 edges at (5.1467, 0, 20.6164)
sketch "Sketch7" plane through (0, 28, 0) normal (0, 1, 0) x (-1, 0, 0)
  line L0 (0, 65) -> (-35, 65)
  line L1 (-35, 65) -> (-35, 0)
  line L2 (-35, 0) -> (0, 0)
  line L3 (0, 0) -> (0, 65)
  line L4 (-30, 15.8253) -> (-23.75, 26.6506)
  line L5 (-23.75, 26.6506) -> (-11.25, 26.6506)
  line L6 (-11.25, 26.6506) -> (-5, 15.8253)
  line L7 (-5, 15.8253) -> (-11.25, 5)
  line L8 (-11.25, 5) -> (-23.75, 5)
  line L9 (-23.75, 5) -> (-30, 15.8253)
  circle A0 centre (-17.5, 15.825) radius 13.25
  dimension "d48" = 26.5
  dimension "d49" = 15.825
  measures "d48" diameter of A0
  measures "d49" distance of L2 A0.centre
extrude "Extrude7" add sketch "Sketch7" along normal blind 1 contours A0
fillet "Fillet3" radius 1 1 edges at (29.8533, 28, 20.6164)
equation "d4 = d1 / 2"

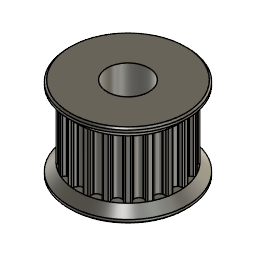
design "GT2-20 idler"
Autodesk Fusion 360 part; units mm, degrees
sketch "Pulley Cylinder" plane through (0, 0, 0) normal (0, 0, 1) x (1, 0, 0) in component "Component"
  circle A0 centre (0, 0) radius 6.1122
extrude "Extrude1" add sketch "Pulley Cylinder" along normal blind 7 in component "Component"
ref_plane "WorkPlane1" through (0, 0, 7) normal (0, 0, 1) x (1, 0, 0) in component "Component"
sketch "Sketch2" plane through (0, 0, 7) normal (0, 0, 1) x (1, 0, 0) in component "Component"
  circle A0 centre (0, 0) radius 7.1122
ref_plane "WorkPlane2" through (0, 0, 0) normal (0, 0, 1) x (1, 0, 0) in component "Component"
sketch "Sketch3" plane through (0, 0, 0) normal (0, 0, 1) x (1, 0, 0) in component "Component"
  circle A0 centre (0, 0) radius 7.1122
extrude "Extrude2" add sketch "Sketch2" along normal blind 1.5 in component "Component"
extrude "Extrude3" add sketch "Sketch3" against normal blind 1.5 in component "Component"
chamfer "Chamfer1" distance 1 angle 45 1 edges at (-6.6309, -2.5719, 0) in component "Component"
chamfer "Chamfer2" distance 1 angle 45 1 edges at (-6.6309, -2.5719, 7) in component "Component"
chamfer "Chamfer3" distance 0.2 angle 45 1 edges at (-6.6309, 2.5719, -1.5) in component "Component"
chamfer "Chamfer4" distance 0.2 angle 45 1 edges at (-6.6309, -2.5719, 8.5) in component "Component"
sketch "Bore" plane through (0, 0, 0) normal (0, 0, 1) x (1, 0, 0) in component "Component"
  circle A0 centre (0, 0) radius 2.5
  constraint coincident A0.centre origin
extrude "Extrude4" cut sketch "Bore" along normal blind 8.5 and the other way blind 1.5 in component "Component"
sketch "Tooth Profile" plane through (0, 0, 0) normal (0, 0, 1) x (1, 0, 0) in component "Component"
  circle A0 centre (0, 0) radius 6.1122 construction
  line L0 (-9.1683, 0) -> (9.1683, 0) construction
  line L1 (6.1122, -6.1122) -> (6.1122, 6.1122) construction
  line L2 (5.1981, 0.4143) -> (6.0981, 0.4143) construction
  line L3 (5.1981, -0.4143) -> (6.0981, -0.4143) construction
  arc A1 (5.5489, 0.4143) -> (5.5489, -0.4143) centre (5.9153, 0) ccw
  line L4 (5.3622, 0.4) -> (5.3622, -0.4) construction
  line L5 (5.5489, 0.4143) -> (5.5489, -0.4143) construction
  arc A2 (5.6176, -0.4626) -> (5.9418, -0.5734) centre (6.0981, 0.4143) ccw
  arc A3 (5.9418, 0.5734) -> (5.6176, 0.4626) centre (6.0981, -0.4143) ccw
  arc A4 (5.9418, 0.5734) -> (6.0673, 0.7397) centre (5.9184, 0.7215) ccw
  arc A5 (5.6176, 0.4626) -> (5.5489, 0.4143) centre (5.799, 0.1316) ccw
  arc A6 (6.0673, -0.7397) -> (5.9418, -0.5734) centre (5.9184, -0.7215) ccw
  arc A7 (5.5489, -0.4143) -> (5.6176, -0.4626) centre (5.799, -0.1316) ccw
  arc A8 (6.0673, -0.7397) -> (6.0673, 0.7397) centre (0, 0) ccw
  point P0 (5.9153, 0)
  point P1 (5.9172, 0)
  point P2 (5.9172, 0)
  dimension "d17" = 12.2244
  dimension "d18" = 0.8287
  dimension "d19" = 0.75
  dimension "d20" = 0.5633
  dimension "d21" = 1
  dimension "d22" = 1
  dimension "d23" = 0.15
  dimension "d24" = 0.15
  constraint coincident A0 L2.end
  constraint coincident A0 L3.end
  constraint coincident A0.centre A8.centre
  constraint midpoint A0.centre L0
  constraint horizontal L0
  constraint vertical L1
  constraint tangent A0 L1
  constraint symmetric L0 L2.start L3.start
  constraint symmetric L0 L2.end L3.end
  constraint horizontal L2
  constraint coincident L2 A1.start
  constraint coincident L3 A1.end
  constraint coincident P0 A1.centre
  constraint symmetric L0 A1.start A1.end
  constraint vertical L4
  constraint tangent A1 L4
  constraint coincident L2.end A2.centre
  constraint coincident L3.end A3.centre
  constraint coincident A0 A4.end
  constraint coincident A3.start A4.start
  constraint tangent A3 A4
  constraint tangent A0 A4
  constraint tangent A1 A5
  constraint coincident A3.end A5.start
  constraint tangent A3 A5
  constraint coincident A0 A6.start
  constraint coincident A2.end A6.end
  constraint tangent A2 A6
  constraint tangent A0 A6
  constraint tangent A1 A7
  constraint coincident A2.start A7.end
  constraint tangent A2 A7
  constraint coincident A4.end A8.end
  measures "d17" diameter of A0
  measures "d18" vertical distance of L2.start L3.start
  measures "d19" horizontal distance of L1.start L4.start
  measures "d20" horizontal distance of L1.start A1.start
  measures "d21" radius of A2
  measures "d22" radius of A3
  measures "d23" radius of A4
  measures "d24" radius of A6
extrude "Extrude5" cut sketch "Tooth Profile" along normal blind 7 in component "Component"
pattern_circular "C-Pattern1" count 20 over 360 about axis through (0, 0, 1.75) along (0, 0, 1) of "Extrude5" in component "Component"
component "Component" placed x (1, 0, 0) y (0, 1, 0) z (0, 0, 1) at (0, 0, 0)
named bodies: "GT2 Pulley"
